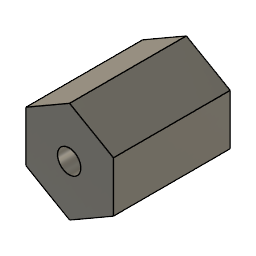
GotekStand (Autodesk Fusion 360 design; units mm, degrees)
Autodesk Fusion 360 part; units mm, degrees
sketch "Sketch1" plane through (0, 0, 0) normal (0, 1, 0) x (1, 0, 0)
  line L0 (3.75, 2.1651) -> (0, 4.3301)
  line L1 (0, 4.3301) -> (-3.75, 2.1651)
  line L2 (-3.75, 2.1651) -> (-3.75, -2.1651)
  line L3 (-3.75, -2.1651) -> (0, -4.3301)
  line L4 (0, -4.3301) -> (3.75, -2.1651)
  line L5 (3.75, -2.1651) -> (3.75, 2.1651)
  dimension "d4" = 3.75
  measures "d4" distance of origin L5
extrude "Extrude1" add sketch "Sketch1" along normal blind 10
hole "Hole1" at (-0.0367, 0, 0.0102) direction (0, 1, 0) diameter 2 depth 10 tip angle 180
